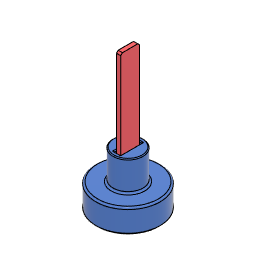
Shutter_Assembly_Param (Autodesk Fusion 360 design; units mm, degrees)
Autodesk Fusion 360 part; units mm, degrees
sketch "Sketch1" plane through (0, 0, 0) normal (0, 1, 0) x (1, 0, 0) in component "Shutter_Cap"
  circle A0 centre (0, 0) radius 3.75
  dimension "d3" = 7.5
  constraint coincident A0.centre origin
  measures "d3" diameter of A0
extrude "Extrude1" add sketch "Sketch1" along normal blind 2.8 makes body 1 in component "Shutter_Cap"
sketch "Sketch2" plane through (0, 2.8, 0) normal (0, 1, 0) x (-1, 0, 0) in component "Shutter_Cap"
  circle A0 centre (0, 0) radius 3.75
  circle A1 centre (0, 0) radius 1.75
  dimension "d8" = 3.5
  constraint coincident A0.centre A1.centre
  measures "d8" diameter of A1
extrude "Extrude2" add sketch "Sketch2" along normal blind 3.5 contours A1 bodies 1 in component "Shutter_Cap"
sketch "Sketch3" plane through (0, 6.3, 0) normal (0, 1, 0) x (-1, 0, 0) in component "Shutter_Cap"
  circle A0 centre (0, 0) radius 1.75
  line L0 (-0.375, 1.25) -> (0.375, 1.25)
  line L1 (0.375, 1.25) -> (0.375, -1.25)
  line L2 (0.375, -1.25) -> (-0.375, -1.25)
  line L3 (-0.375, -1.25) -> (-0.375, 1.25)
  line L4 (-0.375, 1.25) -> (0.375, -1.25) construction
  line L5 (0.375, 1.25) -> (-0.375, -1.25) construction
  dimension "d11" = 0.75
  dimension "d12" = 2.5
  constraint horizontal L0
  constraint perpendicular L0 L1
  constraint parallel L0 L2
  constraint parallel L1 L3
  constraint coincident L4 A0.centre
  constraint coincident L5 A0.centre
  constraint coincident A0.centre origin
  measures "d11" distance of L1.end L2.end
  measures "d12" distance of L0.end L1.end
extrude "Extrude3" cut sketch "Sketch3" against normal blind 2.5 contours L0 L1 L2 L3 bodies 1 in component "Shutter_Cap"
chamfer "Chamfer1" distance 0.2 angle 45 1 edges at (-3.4962, 0, 1.3561) on bodies 1 in component "Shutter_Cap"
chamfer "Chamfer2" distance 0.1 angle 45 1 edges at (1.6316, 6.3, -0.6328) on bodies 1 in component "Shutter_Cap"
fillet "Fillet1" radius 0.2 2 edges at (1.6316, 2.8, 0.6328) (-3.4962, 2.8, 1.3561) on bodies 1 in component "Shutter_Cap"
fillet "Fillet2" radius 0.1 4 edges at (0, 6.3, -1.25) (-0.375, 6.3, 0) (0, 6.3, 1.25) (0.375, 6.3, 0) on bodies 1 in component "Shutter_Cap"
ref_plane "WorkPlane1" through (0, 3.9, 0) normal (0, 1, 0) x (0, 0, 1) in component "Shutter_Blade"
sketch "Sketch1 (2)" plane through (0, 3.9, 0) normal (0, 1, 0) x (1, 0, 0) in component "Shutter_Blade"
  line L0 (0.25, -1.1) -> (-0.25, -1.1)
  line L1 (-0.25, -1.1) -> (-0.25, 1.1)
  line L2 (-0.25, 1.1) -> (0.25, 1.1)
  line L3 (0.25, 1.1) -> (0.25, -1.1)
  line L4 (0.25, -1.1) -> (-0.25, 1.1) construction
  line L5 (-0.25, -1.1) -> (0.25, 1.1) construction
  dimension "d32" = 0.2
  constraint horizontal L0
  constraint perpendicular L0 L1
  constraint parallel L0 L2
  constraint parallel L1 L3
  constraint coincident L4 origin
  constraint coincident L5 origin
  measures "d25" distance of L1.end L2.end
  measures "d26" distance of L0.end L1.end
extrude "Extrude1'" add sketch "Sketch1 (2)" along normal blind 12.5 separate body makes body 2 in component "Shutter_Blade"
chamfer "Chamfer1'" distance 0.2 angle 45 4 edges at (0, 16.4, 1.1) (0, 16.4, -1.1) (0, 3.9, 1.1) (0, 3.9, -1.1) on bodies 2 in component "Shutter_Blade"
component "Shutter_Cap" placed x (1, 0, 0) y (0, 1, 0) z (0, 0, 1) at (0, 0, 0)
component "Shutter_Blade" placed x (1, 0, 0) y (0, 1, 0) z (0, 0, 1) at (0, 0, 0)
equation "Shutter_Cap_Head_Dia = 7.5 mm"
equation "Shutter_Cap_Head_Thk = 2.8 mm"
equation "d3 = Shutter_Cap_Head_Dia"
equation "d4 = Shutter_Cap_Head_Thk"
equation "Shutter_Cap_Shaft_Dia = 3.5 mm"
equation "Shutter_Cap_Shaft_Length = 3.5 mm"
equation "d8 = Shutter_Cap_Shaft_Dia"
equation "d9 = Shutter_Cap_Shaft_Length"
equation "d11 = Shutter_Cap_Slot_W"
equation "d12 = Shutter_Cap_Slot_L"
equation "d13 = -Shutter_Cap_Slot_D"
equation "Shutter_Cap_Slot_W = 0.75 mm"
equation "Shutter_Cap_Slot_L = 2.5 mm"
equation "Shutter_Cap_Slot_D = 2.5 mm"
equation "d25 = Shutter_Blade_W"
equation "d26 = Shutter_Blade_D"
equation "Shutter_Blade_W = 0.5 mm"
equation "Shutter_Blade_D = 2.2 mm"
equation "Shutter_Blade_L = 12.5 mm"
equation "d30 = Shutter_Blade_L"
